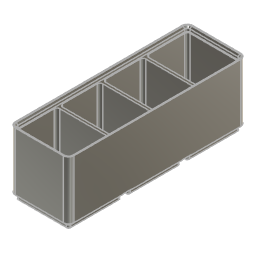
Gridfinity-Sample-Size (Autodesk Fusion 360 design; units mm, degrees)
Autodesk Fusion 360 part; units mm, degrees
ref_plane "WorkPlane1" through (0, 0, 0) normal (0, 0, 1) x (1, 0, 0) in component "Gridfinity bin 3x1x6"
sketch "Base plate sketch" plane through (0, 0, 0) normal (0, 0, 1) x (1, 0, 0) in component "Gridfinity bin 3x1x6"
  line L0 (-0.25, -0.25) -> (41.75, -0.25)
  line L1 (41.75, -0.25) -> (41.75, 41.75)
  line L2 (41.75, 41.75) -> (-0.25, 41.75)
  line L3 (-0.25, 41.75) -> (-0.25, -0.25)
  dimension "d2" = 0.25
  dimension "d3" = 0.25
  dimension "d4" = 42
  dimension "d5" = 42
  constraint horizontal L0
  constraint vertical L1
  constraint horizontal L2
  constraint vertical L3
  measures "d2" vertical distance of origin L0.start
  measures "d3" horizontal distance of origin L2.end
  measures "d4" horizontal distance of L0.start L0.end
  measures "d5" vertical distance of L0.end L1.end
extrude "Base top section extrude" add sketch "Base plate sketch" against normal blind 2.4 makes body 1 in component "Gridfinity bin 3x1x6"
fillet "Base corner fillet" radius 4 8 edges at (-0.25, -0.25, -1.2) (41.75, -0.25, -1.2) (41.75, -0.25, -1.2) (41.75, 41.75, -1.2) (41.75, 41.75, -1.2) (-0.25, 41.75, -1.2) (-0.25, 41.75, -1.2) (-0.25, -0.25, -1.2) on bodies 1 in component "Gridfinity bin 3x1x6"
chamfer "Chamfer1" distance 2.4 angle 45 8 edges at (0.9216, 40.5784, -2.4) (-0.25, 20.75, -2.4) (0.9216, 0.9216, -2.4) (20.75, -0.25, -2.4) (40.5784, 0.9216, -2.4) (41.75, 20.75, -2.4) (40.5784, 40.5784, -2.4) (20.75, 41.75, -2.4) on bodies 1 in component "Gridfinity bin 3x1x6"
extrude "Extrude2" add 1 faces at (15.6168, 15.0833, -2.4) along direction (0, 0, -1) blind 2.6 on bodies 1 bodies 1 in component "Gridfinity bin 3x1x6"
chamfer "Chamfer2" distance 0.8 angle 45 8 edges at (2.6186, 38.8814, -5) (20.75, 39.35, -5) (38.8814, 38.8814, -5) (39.35, 20.75, -5) (38.8814, 2.6186, -5) (20.75, 2.15, -5) (2.6186, 2.6186, -5) (2.15, 20.75, -5) on bodies 1 in component "Gridfinity bin 3x1x6"
pattern_linear "R-Pattern1" count 1 spacing 42 along (1, 0, 0) count 3 spacing 42 along (0, 1, 0) of bodies 1 makes body 2 at (26.4167, 55.75, 0) makes body 3 at (26.4167, 97.75, 0) in component "Gridfinity bin 3x1x6"
sketch "Simple box sketch" plane through (0, 0, 0) normal (0, 0, 1) x (1, 0, 0) in component "Gridfinity bin 3x1x6"
  line L0 (0, 0) -> (41.5, 0)
  line L1 (41.5, 0) -> (41.5, 125.5)
  line L2 (41.5, 125.5) -> (0, 125.5)
  line L3 (0, 125.5) -> (0, 0)
  dimension "d18" = 41.5
  dimension "d19" = 125.5
  constraint horizontal L0
  constraint vertical L1
  constraint horizontal L2
  constraint vertical L3
  constraint coincident L0.start L3
  constraint coincident L3.end L0
  measures "d18" horizontal distance of L0.start L0.end
  measures "d19" vertical distance of L0.end L1.end
extrude "Simple box extrude" add sketch "Simple box sketch" along normal blind 37 separate body makes body 4 in component "Gridfinity bin 3x1x6"
fillet "Bin body corner fillets" radius 3.75 8 edges at (0, 125.5, 18.5) (41.5, 125.5, 18.5) (41.5, 125.5, 18.5) (41.5, 0, 18.5) (41.5, 0, 18.5) (0, 0, 18.5) (0, 0, 18.5) (0, 125.5, 18.5) on bodies 4 in component "Gridfinity bin 3x1x6"
ref_plane "WorkPlane2" through (0, 0, 37) normal (0, 0, 1) x (1, 0, 0) in component "Gridfinity bin 3x1x6"
sketch "Simple box at point sketch" plane through (0, 0, 37) normal (0, 0, 1) x (1, 0, 0) in component "Gridfinity bin 3x1x6"
  line L0 (0, 0) -> (41.5, 0)
  line L1 (41.5, 0) -> (41.5, 125.5)
  line L2 (41.5, 125.5) -> (0, 125.5)
  line L3 (0, 125.5) -> (0, 0)
  dimension "d25" = 41.5
  dimension "d26" = 125.5
  constraint horizontal L0
  constraint vertical L1
  constraint horizontal L2
  constraint vertical L3
  constraint coincident L0.start L3
  constraint coincident L3.end L0
  measures "d25" horizontal distance of L0.start L0.end
  measures "d26" vertical distance of L0.end L1.end
extrude "Simple box at point extrude" add sketch "Simple box at point sketch" along normal blind 4.4 separate body makes body 5 in component "Gridfinity bin 3x1x6"
fillet "Lip body corner fillets" radius 3.75 8 edges at (0, 125.5, 39.2) (41.5, 125.5, 39.2) (41.5, 125.5, 39.2) (41.5, 0, 39.2) (41.5, 0, 39.2) (0, 0, 39.2) (0, 0, 39.2) (0, 125.5, 39.2) on bodies 5 in component "Gridfinity bin 3x1x6"
ref_plane "WorkPlane3" through (0, 0, 42) normal (0, 0, 1) x (1, 0, 0) in component "Gridfinity bin 3x1x6"
sketch "Base plate sketch (1)" plane through (0, 0, 42) normal (0, 0, 1) x (1, 0, 0) in component "Gridfinity bin 3x1x6"
  line L0 (-0.5, -0.5) -> (42, -0.5)
  line L1 (42, -0.5) -> (42, 126)
  line L2 (42, 126) -> (-0.5, 126)
  line L3 (-0.5, 126) -> (-0.5, -0.5)
  dimension "d32" = 0.5
  dimension "d33" = 0.5
  dimension "d34" = 42.5
  dimension "d35" = 126.5
  constraint horizontal L0
  constraint vertical L1
  constraint horizontal L2
  constraint vertical L3
  measures "d32" vertical distance of origin L0.start
  measures "d33" horizontal distance of origin L2.end
  measures "d34" horizontal distance of L0.start L0.end
  measures "d35" vertical distance of L0.end L1.end
extrude "Base top section extrude (1)" add sketch "Base plate sketch (1)" against normal blind 2.4 separate body makes body 6 in component "Gridfinity bin 3x1x6"
fillet "Base corner fillet (1)" radius 4.25 8 edges at (-0.5, -0.5, 40.8) (42, -0.5, 40.8) (42, -0.5, 40.8) (42, 126, 40.8) (42, 126, 40.8) (-0.5, 126, 40.8) (-0.5, 126, 40.8) (-0.5, -0.5, 40.8) on bodies 6 in component "Gridfinity bin 3x1x6"
chamfer "Chamfer3" distance 2.4 angle 45 8 edges at (0.7448, 124.7552, 39.6) (-0.5, 62.75, 39.6) (0.7448, 0.7448, 39.6) (20.75, -0.5, 39.6) (40.7552, 0.7448, 39.6) (42, 62.75, 39.6) (40.7552, 124.7552, 39.6) (20.75, 126, 39.6) on bodies 6 in component "Gridfinity bin 3x1x6"
extrude "Extrude6" add 1 faces at (27.0335, 43.0833, 39.6) along direction (0, 0, -1) blind 2.6 on bodies 6 bodies 6 in component "Gridfinity bin 3x1x6"
ref_plane "WorkPlane4" through (20.75, 62.75, 41.4) normal (0, 0, 1) x (1, 0, 0) in component "Gridfinity bin 3x1x6"
sketch "Lip top chamfer" plane through (0, 0, 41.4) normal (0, 0, 1) x (1, 0, 0) in component "Gridfinity bin 3x1x6"
  line L0 (0, 0) -> (41.5, 0)
  line L1 (41.5, 0) -> (41.5, 125.5)
  line L2 (41.5, 125.5) -> (0, 125.5)
  line L3 (0, 125.5) -> (0, 0)
  dimension "d44" = 41.5
  dimension "d45" = 125.5
  constraint horizontal L0
  constraint vertical L1
  constraint horizontal L2
  constraint vertical L3
  constraint coincident L0.start L3
  constraint coincident L3.end L0
  measures "d44" horizontal distance of L0.start L0.end
  measures "d45" vertical distance of L0.end L1.end
extrude "Lip top chamfer cut" add sketch "Lip top chamfer" against normal blind 0.6 separate body makes body 7 in component "Gridfinity bin 3x1x6"
combine "Combine1" operation cut target body 5 tool bodies 7 6 in component "Gridfinity bin 3x1x6"
ref_plane "WorkPlane5" through (0, 0, 37) normal (0, 0, 1) x (1, 0, 0) in component "Gridfinity bin 3x1x6"
sketch "Simple box at point sketch (1)" plane through (0, 0, 37) normal (0, 0, 1) x (1, 0, 0) in component "Gridfinity bin 3x1x6"
  line L0 (1.2, 1.2) -> (40.3, 1.2)
  line L1 (40.3, 1.2) -> (40.3, 124.3)
  line L2 (40.3, 124.3) -> (1.2, 124.3)
  line L3 (1.2, 124.3) -> (1.2, 1.2)
  dimension "d49" = 1.2
  dimension "d50" = 1.2
  dimension "d51" = 39.1
  dimension "d52" = 123.1
  constraint horizontal L0
  constraint vertical L1
  constraint horizontal L2
  constraint vertical L3
  measures "d49" vertical distance of origin L0.start
  measures "d50" horizontal distance of origin L2.end
  measures "d51" horizontal distance of L0.start L0.end
  measures "d52" vertical distance of L0.end L1.end
extrude "Lip bottom chamfer extrude" add sketch "Simple box at point sketch (1)" along normal blind 2.55 separate body makes body 8 in component "Gridfinity bin 3x1x6"
fillet "Fillet5" radius 2.55 8 edges at (1.2, 124.3, 38.275) (40.3, 124.3, 38.275) (1.2, 1.2, 38.275) (1.2, 124.3, 38.275) (40.3, 124.3, 38.275) (40.3, 1.2, 38.275) (40.3, 1.2, 38.275) (1.2, 1.2, 38.275) on bodies 8 in component "Gridfinity bin 3x1x6"
chamfer "Chamfer4" distance 2.55 angle 45 8 edges at (1.9469, 1.9469, 39.55) (20.75, 1.2, 39.55) (39.5531, 1.9469, 39.55) (40.3, 62.75, 39.55) (39.5531, 123.5531, 39.55) (20.75, 124.3, 39.55) (1.9469, 123.5531, 39.55) (1.2, 62.75, 39.55) on bodies 8 in component "Gridfinity bin 3x1x6"
combine "Combine2" operation cut target body 5 tool bodies 8 in component "Gridfinity bin 3x1x6"
combine "Combine3" operation add target body 4 tool bodies 5 in component "Gridfinity bin 3x1x6"
ref_plane "WorkPlane6" through (0, 0, 0) normal (0, 0, 1) x (1, 0, 0) in component "Gridfinity bin 3x1x6"
sketch "Base clearance cut sketch" plane through (0, 0, 0) normal (0, 0, 1) x (1, 0, 0) in component "Gridfinity bin 3x1x6"
  line L0 (3.75, 0) -> (37.75, 0)
  line L1 (41.5, 3.75) -> (41.5, 121.75)
  line L2 (37.75, 125.5) -> (3.75, 125.5)
  line L3 (0, 121.75) -> (0, 3.75)
  arc A0 (37.75, 0) -> (41.5, 3.75) centre (37.75, 3.75) ccw
  arc A1 (41.5, 121.75) -> (37.75, 125.5) centre (37.75, 121.75) ccw
  arc A2 (3.75, 125.5) -> (0, 121.75) centre (3.75, 121.75) ccw
  arc A3 (0, 3.75) -> (3.75, 0) centre (3.75, 3.75) ccw
  arc A4 (37.75, -10) -> (51.5, 3.75) centre (37.75, 3.75) ccw
  line L4 (51.5, 3.75) -> (51.5, 121.75)
  arc A5 (51.5, 121.75) -> (37.75, 135.5) centre (37.75, 121.75) ccw
  line L5 (37.75, 135.5) -> (3.75, 135.5)
  arc A6 (3.75, 135.5) -> (-10, 121.75) centre (3.75, 121.75) ccw
  line L6 (-10, 121.75) -> (-10, 3.75)
  arc A7 (-10, 3.75) -> (3.75, -10) centre (3.75, 3.75) ccw
  line L7 (3.75, -10) -> (37.75, -10)
  point P0 (41.5, 0)
  point P1 (41.5, 125.5)
  dimension "d59" = 41.5
  dimension "d60" = 125.5
  dimension "d61" = 3.75
  dimension "d62" = 10
  constraint horizontal L0
  constraint vertical L1
  constraint horizontal L2
  constraint vertical L3
  constraint coincident origin L3
  constraint coincident origin L0
  constraint coincident P0 L0
  constraint coincident P0 L1
  constraint tangent L0 A0
  constraint tangent L1 A0
  constraint coincident P1 L1
  constraint coincident P1 L2
  constraint tangent L1 A1
  constraint tangent L2 A1
  constraint tangent L2 A2
  constraint tangent L3 A2
  constraint tangent L3 A3
  constraint tangent L0 A3
  constraint equal A0 A1
  constraint equal A1 A2
  constraint equal A2 A3
  measures "d59" horizontal distance of origin P0
  measures "d60" vertical distance of P0 P1
  measures "d61" radius of A0
extrude "Base side clearance cut" cut sketch "Base clearance cut sketch" along normal blind 1000 and the other way blind 1000 bodies 1 2 3 4 in component "Gridfinity bin 3x1x6"
combine "Combine4" operation add target body 4 tool bodies 2 3 1 1 in component "Gridfinity bin 3x1x6"
sketch "Sketch8" plane through (0, 0, 37) normal (0, 0, 1) x (-1, 0, 0) in component "Gridfinity bin 3x1x6"
  line L0 (-3.75, -1.2) -> (-37.75, -1.2)
  arc A0 (-37.75, -1.2) -> (-40.3, -3.75) centre (-37.75, -3.75) ccw
  line L1 (-40.3, -3.75) -> (-40.3, -121.75)
  arc A1 (-40.3, -121.75) -> (-37.75, -124.3) centre (-37.75, -121.75) ccw
  line L2 (-37.75, -124.3) -> (-3.75, -124.3)
  arc A2 (-3.75, -124.3) -> (-1.2, -121.75) centre (-3.75, -121.75) ccw
  line L3 (-1.2, -121.75) -> (-1.2, -3.75)
  arc A3 (-1.2, -3.75) -> (-3.75, -1.2) centre (-3.75, -3.75) ccw
  line L4 (-1.9, -121.75) -> (-1.9, -3.75)
  arc A4 (-1.9, -3.75) -> (-3.75, -1.9) centre (-3.75, -3.75) ccw
  line L5 (-3.75, -1.9) -> (-37.75, -1.9)
  arc A5 (-37.75, -1.9) -> (-39.6, -3.75) centre (-37.75, -3.75) ccw
  line L6 (-39.6, -3.75) -> (-39.6, -121.75)
  arc A6 (-39.6, -121.75) -> (-37.75, -123.6) centre (-37.75, -121.75) ccw
  line L7 (-37.75, -123.6) -> (-3.75, -123.6)
  arc A7 (-3.75, -123.6) -> (-1.9, -121.75) centre (-3.75, -121.75) ccw
  line L8 (-1.9, -31.375) -> (-39.6, -31.375)
  line L9 (-1.9, -33.275) -> (-39.6, -33.275)
  line L10 (-1.9, -61.8) -> (-39.6, -61.8)
  line L11 (-1.9, -63.7) -> (-39.6, -63.7)
  line L12 (-1.9, -92.225) -> (-39.6, -92.225)
  line L13 (-1.9, -94.125) -> (-39.6, -94.125)
extrude "Extrude10" cut sketch "Sketch8" against normal blind 36 contours L4 L6 A6 L7 A7 L13 | L4 L6 L11 L12 | L4 L6 L9 L10 | L4 A4 L5 A5 L6 L8 bodies 4 in component "Gridfinity bin 3x1x6"
fillet "Fillet6" radius 2 6 edges at (1.9, 94.125, 19) (1.9, 63.7, 19) (1.9, 33.275, 19) (1.9, 61.8, 19) (1.9, 92.225, 19) (1.9, 31.375, 19) on bodies 4 in component "Gridfinity bin 3x1x6"
component "Gridfinity bin 3x1x6" placed x (1, 0, 0) y (0, 1, 0) z (0, 0, 1) at (0, 0, 0)
equation "d6 = -( 2.40 mm )"
equation "d36 = -( 2.40 mm )"
equation "d46 = -( 0.60 mm )"
named bodies: "Base", "Base (1)", "Base (2)", "Gridfinity bin 3x1x6", "Lip body", "Lip cutout"
